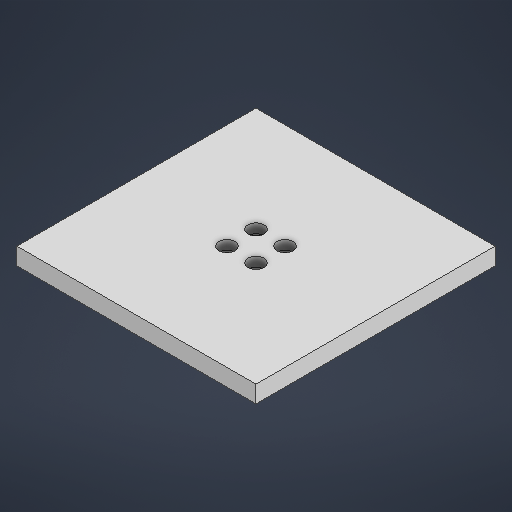
# Autodesk Inventor part: SAL-33 to Saddle Powerbox Adapter-CNC-Anchor-Jig
Saved by Autodesk Inventor 2026.2 (Build 302298010, 298A)
## iProperties
Created: 2026-06-24
Part Number: SAL-33 to Saddle Powerbox Adapter-CNC-Anchor-Jig
Material: Generic
Document SubType Name: Modeling
Designer: incep
Density: 1 g/cm^3
Appearance: Default
Author: incep
## iProperties of the stored document SAL-33 to Saddle Powerbox Adapter-CNC-Anchor-Jig_3DPrint.ipt
Created: 2026-06-24
Part Number: SAL-33 to Saddle Powerbox Adapter-CNC-Anchor-Jig_3DPrint
Material: Generic
Document SubType Name: Modeling
Designer: incep
Density: 1 g/cm^3
Appearance: Default
Author: incep
Autodesk Inventor part; units mm, degrees
ref_plane "YZ Plane" through (0, 0, 0) normal (1, 0, 0) x (0, 1, 0)
ref_plane "XZ Plane" through (0, 0, 0) normal (0, 1, 0) x (-1, 0, 0)
ref_plane "XY Plane" through (0, 0, 0) normal (0, 0, 1) x (1, 0, 0)
sketch "Sketch1" plane through (0, 0, 0) normal (0, 1, 0) x (-1, 0, 0)
  line L0 (0, -140) -> (-140, -140)
  line L1 (-140, -140) -> (-140, 0)
  line L2 (-140, 0) -> (0, 0)
  line L3 (0, 0) -> (0, -140)
  line L4 (-61.5, -78.5) -> (-78.5, -78.5) construction
  line L5 (-78.5, -78.5) -> (-78.5, -61.5) construction
  line L6 (-78.5, -61.5) -> (-61.5, -61.5) construction
  line L7 (-61.5, -61.5) -> (-61.5, -78.5) construction
  circle A0 centre (-61.5, -78.5) radius 2.65
  circle A1 centre (-78.5, -78.5) radius 2.65
  circle A2 centre (-78.5, -61.5) radius 2.65
  circle A3 centre (-61.5, -61.5) radius 2.65
  point P0 (-78.5, -70)
  point P1 (-140, -70)
  point P2 (-70, -78.5)
  point P3 (-70, -140)
  dimension "d0" = 140
  dimension "d1" = 17
  dimension "d2" = 5.3
  constraints: 16 end point, 5 coincident, 4 centre point, 4 midpoint, 4 parallel, 4 perpendicular, 3 equal radius, 2 horizontal, 1 horizontal alignment, 1 vertical alignment
  measures "d0" distance of L2.end L0.start
  measures "d1" distance of L4.start L4.end
  measures "d2" diameter of A0
extrude "Extrusion1" add sketch "Sketch1" along normal blind 10
sketch "Sketch2" plane through (0, 10, 0) normal (0, 1, 0) x (1, 0, 0)
  line L0 (0, 0) -> (140, 0) projected
  line L1 (140, 0) -> (140, 140) projected
  line L2 (140, 140) -> (0, 140) projected
  line L3 (0, 140) -> (0, 0) projected
  circle A0 centre (61.5, 61.5) radius 2.65 projected
  circle A1 centre (78.5, 61.5) radius 2.65 projected
  circle A2 centre (78.5, 78.5) radius 2.65 projected
  circle A3 centre (61.5, 78.5) radius 2.65 projected
  circle A4 centre (61.5, 78.5) radius 4.75
  circle A5 centre (78.5, 78.5) radius 4.75
  circle A6 centre (78.5, 61.5) radius 4.75
  circle A7 centre (61.5, 61.5) radius 4.75
  dimension "d5" = 9.5
  constraints: 4 centre point, 4 coincident, 3 equal radius
  measures "d5" diameter of A4
extrude "Extrusion2" cut sketch "Sketch2" against normal blind 5.5 contours A0 | A1 | A2 | A3 | A4 | A5 | A6 | A7
body "Solid1"
